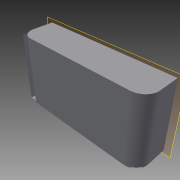
# Autodesk Inventor part: Front
Saved by Autodesk Inventor 2015 SP1 (Build 190203100, 203)
## iProperties
Created: 2015-05-04
Part Number: Front
Material: Generic
Document SubType Name: Modeling
Designer: Brandon
Density: 1 g/cm^3
Appearance: Default
Author: Brandon
Autodesk Inventor part; units mm, degrees
ref_plane "YZ Plane" through (0, 0, 0) normal (1, 0, 0) x (0, 1, 0)
ref_plane "XZ Plane" through (0, 0, 0) normal (0, 1, 0) x (-1, 0, 0)
ref_plane "XY Plane" through (0, 0, 0) normal (0, 0, 1) x (1, 0, 0)
ref_plane "Work Plane1" through (0, 0, 0) normal (0, 0, 1) x (1, 0, 0)
sketch "Sketch1" plane through (0, 0, 0) normal (0, 0, 1) x (1, 0, 0)
  line L0 (-62.5, -32.05) -> (-62.5, 32.05) projected
  line L1 (-62.5, 32.05) -> (62.5, 32.05) projected
  line L2 (62.5, 32.05) -> (62.5, -32.05) projected
  line L3 (62.5, -32.05) -> (-62.5, -32.05) projected
  line L4 (-63.5, -33.05) -> (63.5, -33.05) projected
  line L5 (63.5, -33.05) -> (63.5, 33.05) projected
  line L6 (63.5, 33.05) -> (6.35, 33.05) projected
  line L7 (6.35, 33.05) -> (-6.35, 33.05) projected
  line L8 (-6.35, 33.05) -> (-63.5, 33.05) projected
  line L9 (-63.5, 33.05) -> (-63.5, -33.05) projected
  line L10 (-63.5, 33.05) -> (63.5, 33.05)
  line L11 (63.5, 33.05) -> (63.5, -33.05)
  line L12 (63.5, -33.05) -> (-63.5, -33.05)
  line L13 (-63.5, -33.05) -> (-63.5, 33.05)
  point P0 (0, 0)
  constraints: 8 end point, 2 parallel, 1 horizontal, 1 perpendicular
extrude "Extrusion1" add sketch "Sketch1" along normal blind 32.734 contours L0 L1 L2 L3 | L9 L8 L7 L6 L5 L4
shell "Shell1" thickness 1 removed faces 1 at (-21.1667, -11.0167, 0)
fillet "Fillet1" radius 12.7 2 edges at (63.5, 0, 32.734) (-63.5, 0, 32.734)
fillet "Fillet2" radius 12.7 2 edges at (-62.5, 0, 31.734) (62.5, 0, 31.734)
body "Solid1"
